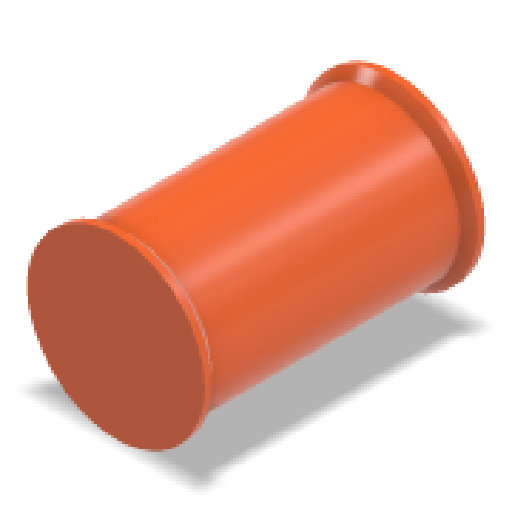
# Autodesk Inventor part: Filament Spool Holder
Saved by Autodesk Inventor 2023.2 (Build 272271000, 271)
## iProperties
Created: 2023-02-25
Part Number: Filament Spool Holder
Material: ABS Plastic
Document SubType Name: Modeling
Designer: remop
Density: 1.06 g/cm^3
Appearance: Smooth - Light Orange
Author: remop
Autodesk Inventor part; units mm, degrees
ref_plane "YZ Plane" through (0, 0, 0) normal (1, 0, 0) x (0, 1, 0)
ref_plane "XZ Plane" through (0, 0, 0) normal (0, 1, 0) x (-1, 0, 0)
ref_plane "XY Plane" through (0, 0, 0) normal (0, 0, 1) x (1, 0, 0)
sketch "Sketch1" plane through (0, 0, 0) normal (0, 0, 1) x (1, 0, 0)
  circle A0 centre (0, 0) radius 22.5
  point P0 (-12.5, 12.5)
  point P1 (12.5, 12.5)
  point P2 (12.5, -12.5)
  point P3 (-12.5, -12.5)
  dimension "d0" = 45
  dimension "d1" = 25
  dimension "d2" = 25
  dimension "d3" = 12.5
  dimension "d4" = 12.5
  constraints: 2 horizontal alignment, 2 vertical alignment, 1 centre point, 1 coincident
  measures "d0" diameter of A0
  measures "d1" distance of point (12.5, 12.5) point (-12.5, 12.5)
  measures "d2" distance of point (12.5, -12.5) point (12.5, 12.5)
  measures "d3" horizontal distance of point (12.5, 12.5) point (0, 0)
  measures "d4" horizontal distance of point (12.5, 12.5) point (0, 0)
extrude "Extrusion1" add sketch "Sketch1" along normal blind 75
sketch "Sketch2" plane through (0, 0, 75) normal (0, 0, 1) x (1, 0, 0)
  circle A0 centre (0, 0) radius 22.5 projected
  circle A1 centre (0, 0) radius 25
  dimension "d7" = 2.5
  constraints: 1 centre point, 1 coincident
  measures "d7" radial gap between concentric circles of A1 A0
extrude "Extrusion2" add sketch "Sketch2" along normal blind 2 contours A0 | A1
chamfer "Chamfer1" distance 2.5 angle 45 1 edges at (-22.5, 0, 75)
sketch "Sketch3" plane through (0, 0, 0) normal (0, 0, -1) x (-1, 0, 0)
  circle A0 centre (0, 0) radius 25 projected
extrude "Extrusion3" add sketch "Sketch3" along normal blind 2
chamfer "Chamfer2" distance 2.5 angle 45 1 edges at (-22.5, 0, 0)
sketch "Sketch4" plane through (0, 0, -2) normal (0, 0, -1) x (-1, 0, 0)
  circle A0 centre (0, 0) radius 25 projected
  point P0 (-12.5, 12.5)
  point P1 (12.5, 12.5)
  point P2 (12.5, -12.5)
  point P3 (-12.5, -12.5)
  dimension "d18" = 12.5
  dimension "d19" = 12.5
  dimension "d20" = 12.5
  dimension "d21" = 12.5
  constraints: 2 horizontal alignment, 2 vertical alignment
  measures "d18" horizontal distance of point (-12.5, 12.5) point (0, 0)
  measures "d19" horizontal distance of point (12.5, 12.5) point (0, 0)
  measures "d20" horizontal distance of point (-12.5, 12.5) point (0, 0)
  measures "d21" horizontal distance of point (0, 0) point (-12.5, -12.5)
hole "Hole1" at (12.5, 12.5, -2) at (-12.5, 12.5, -2) at (-12.5, -12.5, -2) at (12.5, -12.5, -2) direction (0, 0, 1) diameter 2.9 depth 20 tip angle 118
equation "\"d2\" = d1"
equation "\"d3\" = 0.5 * d1"
equation "\"d4\" = d3"
equation "\"d19\" = d18"
equation "\"d20\" = d18"
equation "\"d21\" = d20"
body "Solid1"
